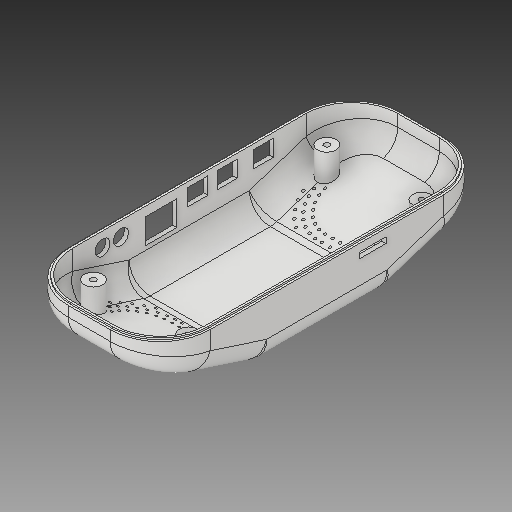
# Autodesk Inventor part: Partie basse
Saved by Autodesk Inventor 2019 (Build 230136000, 136)
## iProperties
Created: 2018-06-04
Part Number: Partie basse
Material: Plastique ABS
Document SubType Name: Modeling
Designer: dimercur
Mass: 82.847 g
Surface Area: 638.157 cm^2
Volume: 78.1576 cm^3
Density: 1.06 g/cm^3
Appearance: Lisse - Blanc
Author: dimercur
Autodesk Inventor part; units mm, degrees
ref_plane "YZ Plane" through (0, 0, 0) normal (1, 0, 0) x (0, 1, 0)
ref_plane "XZ Plane" through (0, 0, 0) normal (0, 1, 0) x (-1, 0, 0)
ref_plane "XY Plane" through (0, 0, 0) normal (0, 0, 1) x (1, 0, 0)
sketch "Esquisse1" plane through (0, 0, 0) normal (0, 1, 0) x (-1, 0, 0)
  line L0 (42.5, 100) -> (-42.5, 100)
  line L1 (-42.5, 100) -> (-42.5, -100)
  line L2 (-42.5, -100) -> (42.5, -100)
  line L3 (42.5, -100) -> (42.5, 100)
  point P0 (0, 0)
  dimension "d0" = 200
  dimension "d1" = 85
  dimension "d2" = 42.5
  dimension "d3" = 100
  constraints: 8 end point, 2 parallel, 1 horizontal, 1 perpendicular
  measures "d0" distance of L2.end L0.start
  measures "d1" distance of L0.start L0.end
  measures "d2" horizontal distance of point (0, 0) L0.start
  measures "d3" vertical distance of point (0, 0) L0.start
extrude "Extrusion1" add sketch "Esquisse1" along normal blind 38
sketch "Esquisse14" plane through (0, 38, 0) normal (0, 1, 0) x (1, 0, 0)
  circle A0 centre (-27.5, -70) radius 3
  circle A1 centre (29.5, -70) radius 3
  circle A2 centre (29.5, 70) radius 3
  circle A3 centre (-27.5, 70) radius 3
  line L0 (-42.5, 100) -> (-42.5, -100) projected
  line L1 (42.5, -100) -> (42.5, 100) projected
  line L2 (-42.5, -100) -> (42.5, -100) projected
  line L3 (42.5, 100) -> (-42.5, 100) projected
  point P0 (0, 0)
  dimension "d110" = 6
  dimension "d111" = 6
  dimension "d112" = 6
  dimension "d113" = 6
  dimension "d114" = 15
  dimension "d115" = 15
  dimension "d116" = 13
  dimension "d117" = 13
  dimension "d118" = 30
  dimension "d119" = 30
  dimension "d120" = 30
  dimension "d121" = 30
  constraints: 4 centre point
  measures "d110" diameter of A0
  measures "d111" diameter of A1
  measures "d112" diameter of A2
  measures "d113" diameter of A3
  measures "d114" distance from line of L0 A0.centre
  measures "d115" distance from line of L0 A3.centre
  measures "d116" distance from line of L1 A1.centre
  measures "d117" distance from line of L1 A2.centre
  measures "d118" distance from line of L2 A0.centre
  measures "d119" distance from line of L2 A1.centre
  measures "d120" distance from line of L3 A3.centre
  measures "d121" distance from line of L3 A2.centre
extrude "Extrusion11" cut sketch "Esquisse14" against normal through all contours A0 | A1 | A2 | A3
chamfer "Chanfrein1" distance 20 angle 72 1 edges at (0, 0, 100) measured on face at (0, 0.5, 100)
chamfer "Chanfrein2" distance 20 angle 72 1 edges at (0, 0, -100) measured on face at (0, 0.5, -100)
fillet "Congé3" radius 30 4 edges at (-42.5, 29, 100) (42.5, 29, 100) (-42.5, 29, -100) (42.5, 29, -100)
fillet "Congé4" radius 15 14 edges at (0, 0, 38.4463) (-33.7132, 17.145, 91.2132) (-42.5, 5.1262, 54.2232) (33.7132, 17.145, 91.2132) (42.5, 5.1262, 54.2232) (0, 20, 100) (-42.5, 0, 0) (42.5, 0, 0) (0, 0, -38.4463) (33.7132, 17.145, -91.2132) (42.5, 5.1262, -54.2232) (-33.7132, 17.145, -91.2132) (-42.5, 5.1262, -54.2232) (0, 20, -100)
shell "Coque1" thickness 2.5 removed faces 1 at (-8.1454, 38, -22.3983)
sketch "Esquisse3" plane through (0, 38, 0) normal (0, 1, 0) x (1, 0, 0)
  arc A0 (42.5, 70) -> (12.5, 100) centre (12.5, 70) ccw projected
  line L0 (12.5, 100) -> (-12.5, 100) projected
  arc A1 (-12.5, 100) -> (-42.5, 70) centre (-12.5, 70) ccw projected
  line L1 (-42.5, 70) -> (-42.5, -70) projected
  arc A2 (-42.5, -70) -> (-12.5, -100) centre (-12.5, -70) ccw projected
  line L2 (-12.5, -100) -> (12.5, -100) projected
  arc A3 (12.5, -100) -> (42.5, -70) centre (12.5, -70) ccw projected
  line L3 (42.5, -70) -> (42.5, 70) projected
  point P0 (0, 0)
extrude "Extrusion2" add sketch "Esquisse3" along normal blind 2.5
sketch "Esquisse4" plane through (0, 40.5, 0) normal (0, 1, 0) x (1, 0, 0)
  line L0 (35, 54) -> (-35, 54)
  line L1 (-35, 54) -> (-35, -54)
  line L2 (-35, -54) -> (35, -54)
  line L3 (35, -54) -> (35, 54)
  line L4 (27.5, -39.9333) -> (-27.5, -39.9333) projected
  circle A0 centre (-18.5, -39.9333) radius 5
  circle A1 centre (-8.5, -80) radius 5
  circle A2 centre (1.5, -39.9333) radius 5
  circle A3 centre (11.5, -80) radius 5
  circle A4 centre (12.5, 78) radius 5
  circle A5 centre (-12.5, 78) radius 5
  circle A6 centre (0.5, 88) radius 5
  circle A7 centre (0.5, 68) radius 5
  line L5 (42.5, -70) -> (42.5, 70) projected
  line L6 (-42.5, 70) -> (-42.5, -70) projected
  line L7 (12.5, 100) -> (-12.5, 100) projected
  line L8 (-12.5, -100) -> (12.5, -100) projected
  point P0 (0, 0)
  dimension "d19" = 108
  dimension "d20" = 70
  dimension "d21" = 35
  dimension "d22" = 54
  dimension "d23" = 10
  dimension "d24" = 10
  dimension "d25" = 10
  dimension "d26" = 10
  dimension "d27" = 10
  dimension "d28" = 10
  dimension "d29" = 10
  dimension "d30" = 10
  dimension "d31" = 25
  dimension "d32" = 12.5
  dimension "d33" = 20
  dimension "d34" = 42
  dimension "d35" = 42
  dimension "d36" = 30
  dimension "d37" = 22
  dimension "d38" = 24
  dimension "d39" = 20
  dimension "d40" = 20
  dimension "d41" = 20
  dimension "d42" = 20
  dimension "d43" = 34
  dimension "d44" = 12
  constraints: 8 centre point, 8 end point, 2 parallel, 2 point on line, 1 horizontal, 1 perpendicular
  measures "d19" distance of L2.end L0.start
  measures "d20" distance of L0.start L0.end
  measures "d21" horizontal distance of point (0, 0) L0.start
  measures "d22" vertical distance of point (0, 0) L0.start
  measures "d23" diameter of A6
  measures "d24" diameter of A4
  measures "d25" diameter of A7
  measures "d26" diameter of A5
  measures "d27" diameter of A2
  measures "d28" diameter of A3
  measures "d29" diameter of A1
  measures "d30" diameter of A0
  measures "d31" distance of A5.centre A4.centre
  measures "d32" horizontal distance of point (0, 0) A4.centre
  measures "d33" distance of A7.centre A6.centre
  measures "d34" distance from line of L5 A6.centre
  measures "d35" distance from line of L5 A7.centre
  measures "d36" distance from line of L6 A5.centre
  measures "d37" distance from line of L7 A4.centre
  measures "d38" distance from line of L6 A0.centre
  measures "d39" distance of A0.centre A2.centre
  measures "d40" distance of A3.centre A1.centre
  measures "d41" distance from line of L8 A1.centre
  measures "d42" distance from line of L8 A3.centre
  measures "d43" distance from line of L6 A1.centre
  measures "d44" distance from line of L7 A6.centre
extrude "Extrusion3" cut sketch "Esquisse4" against normal blind 3 contours L3 L2 L1 L0 | A2 L4 | L4 A2 | A0 L4 | L4 A0 | A1 | A3 | A4 | A5 | A6 | A7
sketch "Esquisse5" plane through (42.5, 15, 36.0706) normal (1, 0, 0) x (0, 0, -1)
  line L0 (-68.9294, 23) -> (139.0706, 23)
  line L1 (139.0706, 23) -> (139.0706, 31)
  line L2 (139.0706, 31) -> (-68.9294, 31)
  line L3 (-68.9294, 31) -> (-68.9294, 23)
  line L4 (-33.9294, 25.5) -> (-63.9294, 25.5) projected
  line L5 (-63.9294, 25.5) -> (-63.9294, 15.8981) projected
  point P0 (36.0706, -15)
  dimension "d47" = 2.5
  dimension "d48" = 208
  dimension "d49" = 5
  dimension "d50" = 8
  constraints: 8 end point, 2 parallel, 1 horizontal, 1 perpendicular
  measures "d47" distance between parallel lines of L0 L4
  measures "d48" distance of L1.end L2.end
  measures "d49" distance between parallel lines of L5 L3
  measures "d50" distance of L2.end L0.start
extrude "Extrusion4" cut sketch "Esquisse5" against normal through all
sketch "Esquisse6" plane through (42.5, 38, 70) normal (0, 1, 0) x (1, 0, 0)
  line L0 (-85, 0) -> (-85, 140) projected
  arc A0 (-85, 0) -> (-55, -30) centre (-55, 0) ccw projected
  line L1 (-30, -30) -> (-55, -30) projected
  arc A1 (-30, -30) -> (0, 0) centre (-30, 0) ccw projected
  line L2 (0, 140) -> (0, 0) projected
  arc A2 (0, 140) -> (-30, 170) centre (-30, 140) ccw projected
  line L3 (-55, 170) -> (-30, 170) projected
  arc A3 (-55, 170) -> (-85, 140) centre (-55, 140) ccw projected
  line L4 (-83.75, 140) -> (-83.75, 0)
  arc A4 (-83.75, 0) -> (-55, -28.75) centre (-55, 0) ccw
  line L5 (-55, -28.75) -> (-30, -28.75)
  arc A5 (-30, -28.75) -> (-1.25, 0) centre (-30, 0) ccw
  line L6 (-1.25, 0) -> (-1.25, 140)
  arc A6 (-1.25, 140) -> (-30, 168.75) centre (-30, 140) ccw
  line L7 (-30, 168.75) -> (-55, 168.75)
  arc A7 (-55, 168.75) -> (-83.75, 140) centre (-55, 140) ccw
  point P0 (-42.5, 70)
  dimension "d53" = 1.25
  constraints: 8 end point, 8 point on circle, 4 centre point, 7 other
  measures "d53" distance between parallel lines of L4 L0
extrude "Extrusion5" cut sketch "Esquisse6" against normal blind 1
sketch "Esquisse7" plane through (0, 0, 0) normal (0, -1, 0) x (1, 0, 0)
  line L0 (-21.7711, -25.1957) -> (-21.7711, 25.1957) construction
  line L1 (-21.7711, 25.1957) -> (-5.7893, 25.1957) construction
  line L2 (-5.7893, 25.1957) -> (-5.7893, -25.1957) construction
  line L3 (-5.7893, -25.1957) -> (-21.7711, -25.1957) construction
  line L4 (8.1956, -14.2694) -> (8.1956, 14.2694) construction
  line L5 (8.1956, 14.2694) -> (25.4477, 14.2694) construction
  line L6 (25.4477, 14.2694) -> (25.4477, -14.2694) construction
  line L7 (25.4477, -14.2694) -> (8.1956, -14.2694) construction
  line L8 (-6.5196, -23.7666) -> (-21.5196, -23.7666)
  line L9 (-21.5196, -23.7666) -> (-21.5196, -20.7369)
  line L10 (-21.5196, -20.7369) -> (-6.5196, -20.7369)
  line L11 (-6.5196, -20.7369) -> (-6.5196, -23.7666)
  line L12 (-6.5196, -17.8215) -> (-21.5196, -17.8215)
  line L13 (-21.5196, -17.8215) -> (-21.5196, -14.8832)
  line L14 (-21.5196, -14.8832) -> (-11.4586, -8.7209)
  line L15 (-11.4586, -8.7209) -> (-21.5196, -8.7209)
  line L16 (-21.5196, -8.7209) -> (-21.5196, -5.9198)
  line L17 (-21.5196, -5.9198) -> (-6.5196, -5.9198)
  line L18 (-6.5196, -5.9198) -> (-6.5196, -8.9496)
  line L19 (-6.5196, -8.9496) -> (-16.3633, -15.0204)
  line L20 (-16.3633, -15.0204) -> (-6.5196, -15.0204)
  line L21 (-6.5196, -15.0204) -> (-6.5196, -17.8215)
  line L22 (-11.4128, -3.4846) -> (-11.6987, -0.5349)
  spline S0 degree 2 poles (-11.6987, -0.5349) (-10.2124, -0.272) (-8.8176, 1.3629) (-8.8176, 2.7349) knots 0 0 0 1 2 2 2
  spline S1 degree 2 poles (-8.8176, 2.7349) (-8.8176, 4.1983) (-10.0523, 5.6846) (-10.8869, 5.6846) knots 0 0 0 1 2 2 2
  spline S2 degree 2 poles (-10.8869, 5.6846) (-11.4243, 5.6846) (-12.1674, 5.0558) (-12.4418, 4.2783) knots 0 0 0 1 2 2 2
  spline S3 degree 2 poles (-12.4418, 4.2783) (-12.6247, 3.7524) (-13.0935, 1.8546) knots 0 0 0 1 1 1
  spline S4 degree 2 poles (-13.0935, 1.8546) (-13.6994, -0.5806) (-14.5798, -1.5639) knots 0 0 0 1 1 1
  spline S5 degree 2 poles (-14.5798, -1.5639) (-15.8145, -2.9473) (-17.5866, -2.9473) knots 0 0 0 1 1 1
  spline S6 degree 2 poles (-17.5866, -2.9473) (-18.7414, -2.9473) (-20.7307, -1.6439) (-21.7711, 0.8027) (-21.7711, 2.5291) knots 0 0 0 1 2 3 3 3
  spline S7 degree 2 poles (-21.7711, 2.5291) (-21.7711, 5.353) (-19.3016, 8.2113) (-17.2322, 8.2799) knots 0 0 0 1 2 2 2
  line L23 (-17.2322, 8.2799) -> (-17.095, 5.2501)
  spline S8 degree 2 poles (-17.095, 5.2501) (-18.2497, 5.0558) (-19.2673, 3.7753) (-19.2673, 2.4948) knots 0 0 0 1 2 2 2
  spline S9 degree 2 poles (-19.2673, 2.4948) (-19.2673, 1.1686) (-18.7299, 0.4254) knots 0 0 0 1 1 1
  spline S10 degree 2 poles (-18.7299, 0.4254) (-18.3755, -0.0547) (-17.7924, -0.0547) knots 0 0 0 1 1 1
  spline S11 degree 2 poles (-17.7924, -0.0547) (-17.2665, -0.0547) (-16.8778, 0.3912) knots 0 0 0 1 1 1
  spline S12 degree 2 poles (-16.8778, 0.3912) (-16.3976, 0.9742) (-15.3572, 5.3988) (-14.2482, 7.5139) (-12.316, 8.7143) (-10.8869, 8.7143) knots 0 0 0 1 2 3 4 4 4
  spline S13 degree 2 poles (-10.8869, 8.7143) (-9.6064, 8.7143) (-7.3542, 7.2852) (-6.2566, 4.6671) (-6.2566, 2.712) knots 0 0 0 1 2 3 3 3
  spline S14 degree 2 poles (-6.2566, 2.712) (-6.2566, -0.1348) (-8.8862, -3.1874) (-11.4128, -3.4846) knots 0 0 0 1 2 2 2
  line L24 (-6.5196, 24.789) -> (-6.5196, 21.4963)
  line L25 (-6.5196, 21.4963) -> (-9.9266, 20.193)
  line L26 (-9.9266, 20.193) -> (-9.9266, 14.2021)
  line L27 (-9.9266, 14.2021) -> (-6.5196, 12.9559)
  line L28 (-6.5196, 12.9559) -> (-6.5196, 9.7433)
  line L29 (-6.5196, 9.7433) -> (-21.5196, 15.5741)
  line L30 (-21.5196, 15.5741) -> (-21.5196, 18.7982)
  line L31 (-21.5196, 18.7982) -> (-6.5196, 24.789)
  line L32 (-12.4647, 19.2212) -> (-18.0211, 17.1518)
  line L33 (-18.0211, 17.1518) -> (-12.4647, 15.1168)
  line L34 (-12.4647, 15.1168) -> (-12.4647, 19.2212)
  line L35 (15.9974, -7.4646) -> (13.9669, -7.4646)
  line L36 (13.9669, -7.4646) -> (13.9669, -2.242)
  line L37 (13.9669, -2.242) -> (18.7413, -2.242)
  spline S15 degree 2 poles (18.7413, -2.242) (19.4822, -3.0011) (20.598, -5.8914) (20.598, -7.3731) knots 0 0 0 1 2 2 2
  spline S16 degree 2 poles (20.598, -7.3731) (20.598, -9.2572) (19.0157, -12.056) (16.0797, -13.4646) (14.3602, -13.4646) knots 0 0 0 1 2 3 3 3
  spline S17 degree 2 poles (14.3602, -13.4646) (12.4852, -13.4646) (9.5675, -11.8914) (8.7901, -10.3822) knots 0 0 0 1 2 2 2
  spline S18 degree 2 poles (8.7901, -10.3822) (8.1956, -9.2207) (8.1956, -7.5011) knots 0 0 0 1 1 1
  spline S19 degree 2 poles (8.1956, -7.5011) (8.1956, -5.2694) (10.0706, -2.7542) (11.7261, -2.3975) knots 0 0 0 1 2 2 2
  line L38 (11.7261, -2.3975) -> (12.1742, -4.803)
  spline S20 degree 2 poles (12.1742, -4.803) (11.287, -5.0591) (10.2627, -6.4585) (10.2627, -7.5011) knots 0 0 0 1 2 2 2
  spline S21 degree 2 poles (10.2627, -7.5011) (10.2627, -9.0926) (12.2749, -10.9676) (14.2596, -10.9676) knots 0 0 0 1 2 2 2
  spline S22 degree 2 poles (14.2596, -10.9676) (16.3907, -10.9676) (18.5309, -9.0652) (18.5309, -7.5286) knots 0 0 0 1 2 2 2
  spline S23 degree 2 poles (18.5309, -7.5286) (18.5309, -6.7694) (17.9364, -5.242) (17.5157, -4.6932) knots 0 0 0 1 2 2 2
  line L39 (17.5157, -4.6932) -> (15.9974, -4.6932)
  line L40 (15.9974, -4.6932) -> (15.9974, -7.4646)
  line L41 (20.3968, -0.0011) -> (8.3968, -0.0011)
  line L42 (8.3968, -0.0011) -> (8.3968, 8.8983)
  line L43 (8.3968, 8.8983) -> (10.4273, 8.8983)
  line L44 (10.4273, 8.8983) -> (10.4273, 2.4226)
  line L45 (10.4273, 2.4226) -> (13.0889, 2.4226)
  line L46 (13.0889, 2.4226) -> (13.0889, 8.4501)
  line L47 (13.0889, 8.4501) -> (15.1194, 8.4501)
  line L48 (15.1194, 8.4501) -> (15.1194, 2.4226)
  line L49 (15.1194, 2.4226) -> (18.3663, 2.4226)
  line L50 (18.3663, 2.4226) -> (18.3663, 9.1269)
  line L51 (18.3663, 9.1269) -> (20.3968, 9.1269)
  line L52 (20.3968, 9.1269) -> (20.3968, -0.0011)
  line L53 (20.3968, 11.1025) -> (8.3968, 11.1025)
  line L54 (8.3968, 11.1025) -> (8.3968, 13.5263)
  line L55 (8.3968, 13.5263) -> (20.3968, 13.5263)
  line L56 (20.3968, 13.5263) -> (20.3968, 11.1025)
  point P0 (0, 0)
  dimension "d56" = 50.3915
  dimension "d57" = 28.5389
  dimension "d59" = 25.1957
  dimension "d60" = 14.2694
  constraints: 4 other
  measures "d56" distance of L0.end L0.start
  measures "d57" distance of L4.end L4.start
  measures "d59" vertical distance of point (0, 0) L0.start
  measures "d60" vertical distance of point (0, 0) L4.start
emboss "Gravure1" sketch "Esquisse7" operation cut depth 1 direction (0, 1, 0)
sketch "Esquisse8" plane through (-42.5, 15, -36.0706) normal (-1, 0, 0) x (0, 0, 1)
  line L0 (43.5706, 17.5) -> (62.0706, 17.5)
  line L1 (62.0706, 17.5) -> (62.0706, 2.5)
  line L2 (62.0706, 2.5) -> (43.5706, 2.5)
  line L3 (43.5706, 2.5) -> (43.5706, 17.5)
  line L4 (136.0706, 15.8981) -> (136.0706, 22) projected
  line L5 (106.0706, 22) -> (-33.9294, 22) projected
  point P0 (36.0706, -15)
  dimension "d64" = 18.5
  dimension "d65" = 15
  dimension "d66" = 74
  dimension "d67" = 19.5
  constraints: 8 end point, 2 parallel, 1 horizontal, 1 perpendicular
  measures "d64" distance of L0.start L0.end
  measures "d65" distance of L0.end L1.end
  measures "d66" distance from line of L4 L0.end
  measures "d67" distance between parallel lines of L2 L5
extrude "Extrusion6" cut sketch "Esquisse8" against normal blind 5
sketch "Esquisse9" plane through (-42.5, 15, -36.0706) normal (-1, 0, 0) x (0, 0, 1)
  circle A0 centre (77.0706, 14.4) radius 4.5
  circle A1 centre (88.0706, 14.4) radius 4.5
  line L0 (106.0706, 22) -> (-33.9294, 22) projected
  point P0 (36.0706, -15)
  point P1 (136.0706, 22)
  dimension "d70" = 9
  dimension "d71" = 9
  dimension "d72" = 48
  dimension "d73" = 59
  dimension "d76" = 7.6
  dimension "d77" = 7.6
  constraints: 2 centre point
  measures "d70" diameter of A0
  measures "d71" diameter of A1
  measures "d72" horizontal distance of point (136.071, 22) A1.centre
  measures "d73" horizontal distance of point (136.071, 22) A0.centre
  measures "d76" distance from line of L0 A0.centre
  measures "d77" vertical distance of point (136.071, 22) A1.centre
extrude "Extrusion7" cut sketch "Esquisse9" against normal blind 5
sketch "Esquisse10" plane through (-42.5, 15, -36.0706) normal (-1, 0, 0) x (0, 0, 1)
  line L0 (-14.4294, 20) -> (-2.4294, 20)
  line L1 (-2.4294, 20) -> (-2.4294, 10)
  line L2 (-2.4294, 10) -> (-14.4294, 10)
  line L3 (-14.4294, 10) -> (-14.4294, 20)
  line L4 (7.3706, 20) -> (19.3706, 20)
  line L5 (19.3706, 20) -> (19.3706, 10)
  line L6 (19.3706, 10) -> (7.3706, 10)
  line L7 (7.3706, 10) -> (7.3706, 20)
  line L8 (24.9706, 20) -> (36.9706, 20)
  line L9 (36.9706, 20) -> (36.9706, 10)
  line L10 (36.9706, 10) -> (24.9706, 10)
  line L11 (24.9706, 10) -> (24.9706, 20)
  line L12 (-63.9294, 22) -> (-63.9294, 15.8981) projected
  line L13 (106.0706, 22) -> (-33.9294, 22) projected
  point P0 (36.0706, -15)
  dimension "d78" = 12
  dimension "d79" = 12
  dimension "d80" = 12
  dimension "d81" = 10
  dimension "d82" = 10
  dimension "d83" = 10
  dimension "d84" = 49.5
  dimension "d85" = 71.3
  dimension "d86" = 88.9
  dimension "d87" = 12
  constraints: 24 end point, 6 parallel, 4 point on line, 3 horizontal, 3 perpendicular
  measures "d78" distance of L0.start L0.end
  measures "d79" distance of L4.start L4.end
  measures "d80" distance of L8.start L8.end
  measures "d81" distance of L2.end L0.start
  measures "d82" distance of L6.end L4.start
  measures "d83" distance of L10.end L8.start
  measures "d84" distance between parallel lines of L12 L3
  measures "d85" distance from line of L12.start L7
  measures "d86" distance between parallel lines of L12 L11
  measures "d87" distance from line of L1.end L13
extrude "Extrusion8" cut sketch "Esquisse10" against normal blind 5
sketch "Esquisse11" plane through (42.5, 15, 36.0706) normal (1, 0, 0) x (0, 0, -1)
  line L0 (55.5706, 17.5) -> (71.5706, 17.5)
  line L1 (71.5706, 17.5) -> (71.5706, 14)
  line L2 (71.5706, 14) -> (55.5706, 14)
  line L3 (55.5706, 14) -> (55.5706, 17.5)
  line L4 (106.0706, 22) -> (-33.9294, 22) projected
  point P0 (36.0706, -15)
  point P1 (136.0706, 22)
  dimension "d90" = 3.5
  dimension "d91" = 16
  dimension "d92" = 4.5
  dimension "d93" = 64.5
  constraints: 8 end point, 2 parallel, 1 horizontal, 1 perpendicular
  measures "d90" distance between parallel lines of L2 L0
  measures "d91" distance of L0.start L0.end
  measures "d92" distance between parallel lines of L4 L0
  measures "d93" distance from line of L1 point (136.071, 22)
extrude "Extrusion9" cut sketch "Esquisse11" against normal blind 5
sketch "Esquisse15" plane through (-27.5, 38, 70) normal (0, 1, 0) x (1, 0, 0)
  circle A0 centre (0, 0) radius 5.5 projected
  circle A1 centre (57, 0) radius 5.5 projected
  circle A2 centre (57, 140) radius 5.5 projected
  circle A3 centre (0, 140) radius 5.5 projected
  point P0 (27.5, 70)
extrude "Extrusion12" cut sketch "Esquisse15" against normal blind 13
sketch "Esquisse16" plane through (-27.5, 25, 70) normal (0, 1, 0) x (1, 0, 0)
  circle A0 centre (0, 0) radius 5.5 projected
  circle A1 centre (57, 0) radius 5.5 projected
  circle A2 centre (57, 140) radius 5.5 projected
  circle A3 centre (0, 140) radius 5.5 projected
  circle A4 centre (0, 0) radius 1.75
  circle A5 centre (57, 0) radius 1.75
  circle A6 centre (57, 140) radius 1.75
  circle A7 centre (0, 140) radius 1.75
  point P0 (27.5, 70)
  dimension "d126" = 3.5
  dimension "d127" = 3.5
  dimension "d128" = 3.5
  dimension "d129" = 3.5
  constraints: 4 centre point, 4 coincident
  measures "d126" diameter of A4
  measures "d127" diameter of A5
  measures "d128" diameter of A6
  measures "d129" diameter of A7
extrude "Extrusion13" add sketch "Esquisse16" along normal blind 3
sketch "Esquisse17" plane through (0, 0, 0) normal (0, -1, 0) x (1, 0, 0)
  line L0 (-79.1178, 0) -> (59.6619, 0)
  circle A0 centre (-4.5, 46) radius 0.75
  line L1 (12.5, 100) -> (-12.5, 100) projected
  circle A1 centre (-4.5, 64) radius 0.5
  line L2 (-42.5, 70) -> (-42.5, 36.0706) projected
  line L3 (0, 119.1841) -> (0, -113.7497)
  line L4 (-42.5, -36.0706) -> (-42.5, -70) projected
  line L5 (-12.5, -100) -> (12.5, -100) projected
  circle A2 centre (-8.5054, 46.4513) radius 0.75
  circle A3 centre (-12.3099, 47.7826) radius 0.75
  circle A4 centre (-15.7228, 49.927) radius 0.75
  circle A5 centre (-18.573, 52.7772) radius 0.75
  circle A6 centre (-20.7174, 56.1901) radius 0.75
  circle A7 centre (-22.0487, 59.9946) radius 0.75
  circle A8 centre (-22.5, 64) radius 0.75
  circle A9 centre (-6.5, 42) radius 0.75
  circle A10 centre (-10.7139, 42.8012) radius 0.75
  circle A11 centre (-14.6936, 44.4018) radius 0.75
  circle A12 centre (-18.2889, 46.7412) radius 0.75
  circle A13 centre (-21.3643, 49.7313) radius 0.75
  circle A14 centre (-23.8039, 53.2594) radius 0.75
  circle A15 centre (-25.5157, 57.1925) radius 0.75
  circle A16 centre (-26.4351, 61.3822) radius 0.75
  circle A17 centre (-18, 42) radius 0.75
  circle A18 centre (-22.0326, 45.0564) radius 0.75
  circle A19 centre (-25.3914, 48.8409) radius 0.75
  circle A20 centre (-27.9474, 53.2079) radius 0.75
  circle A21 centre (-29.6023, 57.9896) radius 0.75
  circle A22 centre (4.5, 46) radius 0.75
  circle A23 centre (4.5, 64) radius 0.5
  circle A24 centre (8.5054, 46.4513) radius 0.75
  circle A25 centre (12.3099, 47.7826) radius 0.75
  circle A26 centre (15.7228, 49.927) radius 0.75
  circle A27 centre (18.573, 52.7772) radius 0.75
  circle A28 centre (20.7174, 56.1901) radius 0.75
  circle A29 centre (22.0487, 59.9946) radius 0.75
  circle A30 centre (22.5, 64) radius 0.75
  circle A31 centre (6.5, 42) radius 0.75
  circle A32 centre (10.7139, 42.8012) radius 0.75
  circle A33 centre (14.6936, 44.4018) radius 0.75
  circle A34 centre (18.2889, 46.7412) radius 0.75
  circle A35 centre (21.3643, 49.7313) radius 0.75
  circle A36 centre (23.8039, 53.2594) radius 0.75
  circle A37 centre (25.5157, 57.1925) radius 0.75
  circle A38 centre (26.4351, 61.3822) radius 0.75
  circle A39 centre (18, 42) radius 0.75
  circle A40 centre (22.0326, 45.0564) radius 0.75
  circle A41 centre (25.3914, 48.8409) radius 0.75
  circle A42 centre (27.9474, 53.2079) radius 0.75
  circle A43 centre (29.6023, 57.9896) radius 0.75
  circle A44 centre (-4.5, -46) radius 0.75
  circle A45 centre (-4.5, -64) radius 0.5
  circle A46 centre (-8.5054, -46.4513) radius 0.75
  circle A47 centre (-12.3099, -47.7826) radius 0.75
  circle A48 centre (-15.7228, -49.927) radius 0.75
  circle A49 centre (-18.573, -52.7772) radius 0.75
  circle A50 centre (-20.7174, -56.1901) radius 0.75
  circle A51 centre (-22.0487, -59.9946) radius 0.75
  circle A52 centre (-22.5, -64) radius 0.75
  circle A53 centre (-6.5, -42) radius 0.75
  circle A54 centre (-10.7139, -42.8012) radius 0.75
  circle A55 centre (-14.6936, -44.4018) radius 0.75
  circle A56 centre (-18.2889, -46.7412) radius 0.75
  circle A57 centre (-21.3643, -49.7313) radius 0.75
  circle A58 centre (-23.8039, -53.2594) radius 0.75
  circle A59 centre (-25.5157, -57.1925) radius 0.75
  circle A60 centre (-26.4351, -61.3822) radius 0.75
  circle A61 centre (-18, -42) radius 0.75
  circle A62 centre (-22.0326, -45.0564) radius 0.75
  circle A63 centre (-25.3914, -48.8409) radius 0.75
  circle A64 centre (-27.9474, -53.2079) radius 0.75
  circle A65 centre (-29.6023, -57.9896) radius 0.75
  circle A66 centre (15.7228, -49.927) radius 0.75
  circle A67 centre (12.3099, -47.7826) radius 0.75
  circle A68 centre (8.5054, -46.4513) radius 0.75
  circle A69 centre (4.5, -46) radius 0.75
  circle A70 centre (18.2889, -46.7412) radius 0.75
  circle A71 centre (14.6936, -44.4018) radius 0.75
  circle A72 centre (25.3914, -48.8409) radius 0.75
  circle A73 centre (10.7139, -42.8012) radius 0.75
  circle A74 centre (6.5, -42) radius 0.75
  circle A75 centre (22.0326, -45.0564) radius 0.75
  circle A76 centre (18, -42) radius 0.75
  circle A77 centre (21.3643, -49.7313) radius 0.75
  circle A78 centre (18.573, -52.7772) radius 0.75
  circle A79 centre (20.7174, -56.1901) radius 0.75
  circle A80 centre (23.8039, -53.2594) radius 0.75
  circle A81 centre (27.9474, -53.2079) radius 0.75
  circle A82 centre (22.0487, -59.9946) radius 0.75
  circle A83 centre (25.5157, -57.1925) radius 0.75
  circle A84 centre (29.6023, -57.9896) radius 0.75
  circle A85 centre (22.5, -64) radius 0.75
  circle A86 centre (26.4351, -61.3822) radius 0.75
  circle A87 centre (4.5, -64) radius 0.5
  circle A88 centre (0, 45.9912) radius 0.75
  circle A89 centre (0, -45.9912) radius 0.75
  circle A90 centre (-2.5, -42) radius 0.75
  circle A91 centre (2.5, -42) radius 0.75
  circle A92 centre (-2.5, 42) radius 0.75
  circle A93 centre (2.5, 42) radius 0.75
  point P0 (0, 0)
  dimension "d134" = 1.5
  dimension "d135" = 54
  dimension "d136" = 36
  dimension "d138" = 42.5
  dimension "d139" = 100
  dimension "d140" = 38
  dimension "d143" = 90
  dimension "d145" = 38
  dimension "d146" = 1
  dimension "d147" = 1.5
  dimension "d148" = 58
  dimension "d149" = 36
  dimension "d152" = 78
  dimension "d154" = 1.5
  dimension "d155" = 24.5
  dimension "d156" = 58
  dimension "d159" = 45
  dimension "d161" = 1.5
  dimension "d163" = 1.5
  dimension "d164" = 1.5
  dimension "d165" = 1.5
  dimension "d166" = 1.5
  dimension "d167" = 1.5
  dimension "d168" = 4
  dimension "d169" = 4
  dimension "d170" = 4
  dimension "d171" = 4
  constraints: 94 centre point, 66 symmetric about line, 4 end point, 2 point on line, 1 horizontal, 1 vertical, 105 other
  measures "d134" diameter of A0
  measures "d135" distance from line of L1 A0.centre
  measures "d136" distance from line of L1 A1.centre
  measures "d138" distance between parallel lines of L4 L3
  measures "d139" distance between parallel lines of L5 L0
  measures "d140" distance from line of L2 A1.centre
  measures "d145" distance from line of L2 A0.centre
  measures "d146" diameter of A1
  measures "d147" diameter of A9
  measures "d148" distance from line of L1 A9.centre
  measures "d149" distance from line of L2 A9.centre
  measures "d154" diameter of A17
  measures "d155" distance from line of L2 A17.centre
  measures "d156" distance from line of L1 A17.centre
  measures "d161" diameter of A88
  measures "d163" diameter of A89
  measures "d164" diameter of A90
  measures "d165" diameter of A91
  measures "d166" diameter of A92
  measures "d167" diameter of A93
  measures "d168" distance of A92.centre A9.centre
  measures "d169" distance of A31.centre A93.centre
  measures "d170" distance of A90.centre A53.centre
  measures "d171" distance of A74.centre A91.centre
extrude "Extrusion14" cut sketch "Esquisse17" against normal through all contours A0 | A88 L3 | L3 A88 | A89 L3 | L3 A89 | A2 | A3 | A4 | A5 | A6 | A7 | A8 | A9 | A10 | A11 | A12 | A13 | A14 | A15 | A16 | A17 | A18 | A19 | A20 | A21 | A22 | A24 | A25 | A26 | A27 | A28 | A29 | A30 | A31 | A32 | A33 | A34 | A35 | A36 | A37 | A38 | A39 | A40 | A41 | A42 | A43 | A44 | A46 | A47 | A48 | A49 | A50 | A51 | A52 | A53 | A54 | A55 | A56 | A57 | A58 | A59 | A60 | A61 | A62 | A63 | A64 | A65 | A66 | A67 | A68 | A69 | A70 | A71 | A72 | A73 | A74 | A75 | A76 | A77 | A78 | A79 | A80 | A81 | A82 | A83 | A84 | A85 | A86 | A90 | A91 | A92 | A93
equation "\"d111\" = d110"
equation "\"d112\" = d110"
equation "\"d113\" = d110"
equation "\"d115\" = d114"
equation "\"d117\" = d116"
equation "\"d118\" = d119"
equation "\"d120\" = d118"
equation "\"d121\" = d119"
equation "\"d2\" = 0.5 * d1"
equation "\"d3\" = 0.5 * d0"
equation "\"d21\" = 0.5 * d20"
equation "\"d22\" = 0.5 * d19"
equation "\"d32\" = 0.5 * d31"
equation "\"d59\" = 0.5 * d56"
equation "\"d60\" = 0.5 * d57"
equation "\"d71\" = d70"
equation "\"d77\" = d76"
equation "\"d79\" = d78"
equation "\"d80\" = d78"
equation "\"d127\" = d126"
equation "\"d128\" = d126"
equation "\"d129\" = d126"
